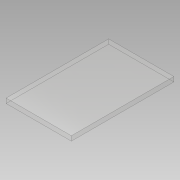
# Autodesk Inventor part: TAPA INFERIOR
Saved by Autodesk Inventor 2019 (Build 230136000, 136)
## iProperties
Created: 2020-04-08
Part Number: TAPA INFERIOR
Material: Plástico PMMA
Document SubType Name: Modeling
Designer: Luis Pujol
Density: 1.188 g/cm^3
Appearance: Policarbonato - Claro
Author: Luis Pujol
Autodesk Inventor part; units mm, degrees
ref_plane "YZ Plane" through (0, 0, 0) normal (1, 0, 0) x (0, 1, 0)
ref_plane "XZ Plane" through (0, 0, 0) normal (0, 1, 0) x (-1, 0, 0)
ref_plane "XY Plane" through (0, 0, 0) normal (0, 0, 1) x (1, 0, 0)
sketch "Boceto1" plane through (0, 0, 0) normal (0, 1, 0) x (-1, 0, 0)
  line L0 (-70, 110) -> (70, 110)
  line L1 (70, 110) -> (70, -110)
  line L2 (70, -110) -> (-70, -110)
  line L3 (-70, -110) -> (-70, 110)
  line L4 (-70, 110) -> (70, -110) construction
  line L5 (70, 110) -> (-70, -110) construction
  point P0 (0, 0)
  dimension "d0" = 140
  dimension "d1" = 220
  constraints: 12 end point, 2 midpoint, 2 parallel, 1 horizontal, 1 perpendicular
  measures "d0" distance of L1.end L2.end
  measures "d1" distance of L0.end L1.end
extrude "Extrusión1" add sketch "Boceto1" along normal blind 10
